Encoder v2 (Autodesk Fusion 360 design; units mm, degrees)
Autodesk Fusion 360 part; units mm, degrees
sketch "Sketch1" plane through (0, 0, 0) normal (0, 0, 1) x (1, 0, 0)
  line L0 (11.5, 11.5) -> (-11.5, 11.5) construction
  line L1 (-11.5, 11.5) -> (-11.5, -11.5) construction
  line L2 (-11.5, -11.5) -> (11.5, -11.5) construction
  line L3 (11.5, -11.5) -> (11.5, 11.5) construction
  line L4 (11.5, 11.5) -> (-11.5, -11.5) construction
  line L5 (-11.5, 11.5) -> (11.5, -11.5) construction
  line L6 (9.7, 9.75) -> (-9.7, 9.75) construction
  line L7 (-9.7, 9.75) -> (-9.7, -9.75) construction
  line L8 (-9.7, -9.75) -> (9.7, -9.75) construction
  line L9 (9.7, -9.75) -> (9.7, 9.75) construction
  line L10 (9.7, 9.75) -> (-9.7, -9.75) construction
  line L11 (-9.7, 9.75) -> (9.7, -9.75) construction
  line L12 (11.5, 6.3) -> (-11.5, 6.3) construction
  line L13 (6.3, 11.5) -> (6.3, -11.5) construction
  line L14 (-11.5, -6.3) -> (11.5, -6.3) construction
  line L15 (-6.3, 11.5) -> (-6.3, -11.5) construction
  line L16 (-11.5, 0) -> (11.5, 0) construction
  line L17 (0, 11.5) -> (0, -11.5) construction
  circle A0 centre (8.025, 8.025) radius 1.725
  circle A1 centre (-8.025, 8.025) radius 1.725
  circle A2 centre (-8.025, -8.025) radius 1.725
  circle A3 centre (7.975, -8.025) radius 1.725
  circle A4 centre (8.025, 8.025) radius 3.475 construction
  circle A5 centre (-8.025, 8.025) radius 3.475 construction
  circle A6 centre (-8.025, -8.025) radius 3.475 construction
  circle A7 centre (7.975, -8.025) radius 3.475 construction
  line L18 (11.5, 8.0142) -> (11.45, -8.0358)
  arc A8 (7.975, -11.5) -> (11.45, -8.0358) centre (7.975, -8.025) ccw
  line L19 (7.975, -11.5) -> (-8.025, -11.5)
  arc A9 (-11.5, -8.025) -> (-8.025, -11.5) centre (-8.025, -8.025) ccw
  line L20 (-11.5, -8.025) -> (-11.5, 8.025)
  arc A10 (-8.025, 11.5) -> (-11.5, 8.025) centre (-8.025, 8.025) ccw
  line L21 (-8.025, 11.5) -> (8.025, 11.5)
  arc A11 (11.5, 8.0142) -> (8.025, 11.5) centre (8.025, 8.025) ccw
  dimension "d1" = 23
  dimension "d2" = 23
  dimension "d3" = 19.4
  dimension "d4" = 19.5
  dimension "d5" = 12.6
  dimension "d6" = 6.3
  dimension "d7" = 6.3
  dimension "d8" = 12.6
  constraint horizontal L0
  constraint perpendicular L0 L1
  constraint parallel L0 L2
  constraint parallel L1 L3
  constraint coincident L4 origin
  constraint coincident L5 origin
  constraint horizontal L6
  constraint perpendicular L6 L7
  constraint parallel L6 L8
  constraint parallel L7 L9
  constraint coincident L10 origin
  constraint coincident L11 origin
  constraint coincident L3 L12.start
  constraint coincident L1 L12.end
  constraint perpendicular L1 L12
  constraint coincident L0 L13.start
  constraint coincident L2 L13.end
  constraint perpendicular L2 L13
  constraint coincident L1 L14.start
  constraint coincident L3 L14.end
  constraint perpendicular L3 L14
  constraint coincident L0 L15.start
  constraint coincident L2 L15.end
  constraint perpendicular L2 L15
  constraint midpoint L1 L16.start
  constraint midpoint L3 L16.end
  constraint midpoint L0 L17.start
  constraint midpoint L2 L17.end
  constraint tangent L12 A0
  constraint tangent L12 A1
  constraint tangent L8 A2
  constraint tangent L8 A3
  constraint tangent L6 A1
  constraint tangent L15 A1
  constraint tangent L6 A0
  constraint tangent L13 A0
  constraint tangent L14 A3
  constraint tangent L9 A3
  constraint tangent L15 A2
  constraint tangent L14 A2
  constraint concentric A0 A4
  constraint tangent L0 A4
  constraint concentric A1 A5
  constraint tangent L0 A5
  constraint concentric A2 A6
  constraint tangent L1 A6
  constraint concentric A3 A7
  constraint tangent L2 A7
  constraint coincident A4 L18.start
  constraint coincident A7 L18.end
  constraint tangent A7 L18
  constraint coincident L2 A8.start
  constraint coincident A7 A8.start
  constraint tangent L18 A8
  constraint coincident L2 L19.end
  constraint coincident A6 L19.end
  constraint coincident A6 A9.start
  constraint tangent L19 A9
  constraint coincident A5 L20.end
  constraint tangent A5 L20
  constraint coincident A5 A10.start
  constraint tangent L20 A10
  constraint coincident A4 L21.end
  constraint tangent A4 L21
  constraint tangent L21 A11
  constraint tangent A4 L18
  measures "d1" distance of L1.end L2.end
  measures "d2" distance of L0.end L1.end
  measures "d3" distance of L7.end L8.end
  measures "d4" distance of L6.end L7.end
  measures "d5" distance of L12 L14
  measures "d6" distance of L12 L16
  measures "d7" distance of L13 L17
  measures "d8" distance of L13 L15
extrude "Extrude1" add sketch "Sketch1" along normal blind 1.6 makes body 1
sketch "Sketch3" plane through (0, 0, 1.6) normal (0, 0, 1) x (-1, 0, 0)
  circle A0 centre (-7.975, 8.025) radius 1.725
  circle A1 centre (8.025, -8.025) radius 1.725
  circle A2 centre (-8.025, -8.025) radius 1.725
  circle A3 centre (8.025, 8.025) radius 1.725
  arc A4 (-7.975, 11.5) -> (-11.45, 8.0358) centre (-7.975, 8.025) ccw
  line L0 (-11.45, 8.0358) -> (-11.5, -8.0142)
  arc A5 (-11.5, -8.0142) -> (-8.025, -11.5) centre (-8.025, -8.025) ccw
  line L1 (-8.025, -11.5) -> (8.025, -11.5)
  arc A6 (8.025, -11.5) -> (11.5, -8.025) centre (8.025, -8.025) ccw
  line L2 (11.5, -8.025) -> (11.5, 8.025)
  arc A7 (11.5, 8.025) -> (8.025, 11.5) centre (8.025, 8.025) ccw
  line L3 (8.025, 11.5) -> (-7.975, 11.5)
  line L4 (-3.5, 3.5) -> (3.5, 3.5)
  line L5 (3.5, 3.5) -> (3.5, -3.5)
  line L6 (3.5, -3.5) -> (-3.5, -3.5)
  line L7 (-3.5, -3.5) -> (-3.5, 3.5)
  line L8 (-3.5, 3.5) -> (3.5, -3.5) construction
  line L9 (3.5, 3.5) -> (-3.5, -3.5) construction
  point P0 (8.025, 8.025)
  point P1 (8.025, 8.025)
  dimension "d15" = 7
  dimension "d16" = 7
  constraint horizontal L4
  constraint perpendicular L4 L5
  constraint parallel L4 L6
  constraint parallel L5 L7
  constraint coincident L8 origin
  constraint coincident L9 origin
  measures "d15" distance of L5.end L6.end
  measures "d16" distance of L4.end L5.end
extrude "Extrude3" add sketch "Sketch3" along normal blind 1.5 separate body contours L4 L5 L6 L7 makes body 2
copy_body "Body->Comp1" bodies 2 removing the originals makes body 3 in component "Sensor"
component "Sensor" placed x (1, 0, 0) y (0, 1, 0) z (0, 0, 1) at (0, 0, 0)
equation "d5 = d6 * 2"
equation "d6 = ( 12.5 / 2 ) * 1 mm + 0.05 mm"
equation "d7 = d6"
equation "d8 = d5"
